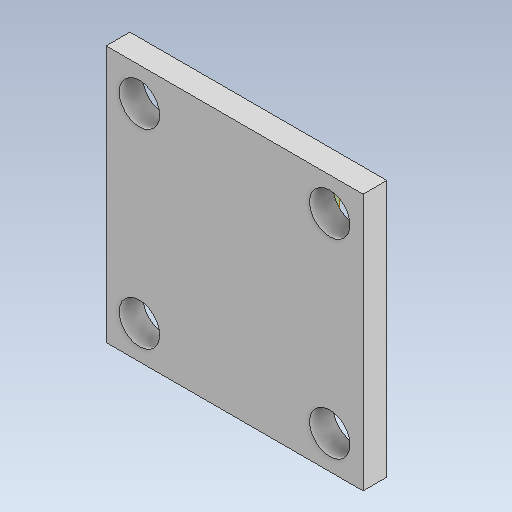
# Autodesk Inventor part: Magazin_1_trichter
Saved by Autodesk Inventor 2025.2 (Build 292293000, 293)
## iProperties
Created: 2025-06-10
Part Number: Magazin_1_trichter
Material: Generisch
Document SubType Name: Modeling
Designer: maria
Density: 1 g/cm^3
Appearance: Vorgabe
Author: maria
## iProperties of the stored document Magazin_1_3D-Druck.ipt
Created: 2025-06-10
Part Number: Magazin_1_3D-Druck
Material: Generisch
Document SubType Name: Modeling
Designer: maria
Density: 1 g/cm^3
Appearance: Vorgabe
Author: maria
Autodesk Inventor part; units mm, degrees
ref_plane "YZ Plane" through (0, 0, 0) normal (1, 0, 0) x (0, 1, 0)
ref_plane "XZ Plane" through (0, 0, 0) normal (0, 1, 0) x (-1, 0, 0)
ref_plane "XY Plane" through (0, 0, 0) normal (0, 0, 1) x (1, 0, 0)
sketch "Skizze1" plane through (0, 0, 0) normal (0, 1, 0) x (-1, 0, 0)
  line L0 (0, 0) -> (12, 0)
  line L1 (12, 0) -> (12, -16)
  line L2 (12, -16) -> (0, -16)
  line L3 (0, -16) -> (0, 0)
  line L4 (17, 5) -> (17, -21)
  line L5 (-5, -21) -> (-5, 5)
  line L6 (-1, 1) -> (13, 1)
  line L7 (13, 1) -> (13, -17)
  line L8 (13, -17) -> (-1, -17)
  line L9 (-1, -17) -> (-1, 1)
  line L10 (1.75, -1.75) -> (10.25, -1.75)
  line L11 (10.25, -1.75) -> (10.25, -14.25)
  line L12 (10.25, -14.25) -> (1.75, -14.25)
  line L13 (1.75, -14.25) -> (1.75, -1.75)
  line L14 (0.75, -0.75) -> (11.25, -0.75)
  line L15 (11.25, -0.75) -> (11.25, -15.25)
  line L16 (11.25, -15.25) -> (0.75, -15.25)
  line L17 (0.75, -15.25) -> (0.75, -0.75)
  line L18 (15.25, 5.25) -> (-3.25, 5.25)
  line L19 (-3.25, 5.25) -> (-3.25, -21.25)
  line L20 (-3.25, -21.25) -> (15.25, -21.25)
  line L21 (15.25, -21.25) -> (15.25, 5.25)
  line L22 (16.25, 6.25) -> (-4.25, 6.25)
  line L23 (-4.25, 6.25) -> (-4.25, -22.25)
  line L24 (-4.25, -22.25) -> (16.25, -22.25)
  line L25 (16.25, -22.25) -> (16.25, 6.25)
  point P0 (6, 0)
  point P1 (6, 5)
  point P2 (6, -16)
  point P3 (12, -8)
  point P4 (6, -1.75)
  point P5 (6, -14.25)
  point P6 (10.25, -8)
  point P7 (1.75, -8)
  point P8 (6, -21.25)
  dimension "d0" = 16
  dimension "d1" = 12
  dimension "d2" = 5
  dimension "d3" = 5
  dimension "d56" = 1
  dimension "d57" = 1
  dimension "d58" = 1
  dimension "d60" = 1.75
  dimension "d61" = 1.75
  dimension "d63" = 8.5
  dimension "d64" = 1
  dimension "d65" = 1
  dimension "d67" = 1
  dimension "d69" = 12.5
  dimension "d70" = 1
  dimension "d71" = 1.75
  dimension "d72" = 1.75
  dimension "d74" = 7
  dimension "d76" = 7
  dimension "d77" = 5
  dimension "d78" = 5
  dimension "d80" = 1
  dimension "d81" = 1
  dimension "d82" = 1
  dimension "d83" = 1
  constraints: 52 end point, 13 parallel, 8 midpoint, 6 horizontal, 6 perpendicular
  measures "d0" distance of L0.end L1.end
  measures "d1" distance of L1.end L2.end
  measures "d2" distance between parallel lines of L4 L1
  measures "d3" distance between parallel lines of L5 L3
  measures "d56" distance between parallel lines of L0 L6
  measures "d57" distance from line of L7 point (12, -8)
  measures "d58" distance between parallel lines of L8 L2
  measures "d60" distance of point (6, 0) point (6, -1.75)
  measures "d61" distance from line of L2 point (6, -14.25)
  measures "d63" distance of point (10.25, -8) point (1.75, -8)
  measures "d64" distance between parallel lines of L10 L14
  measures "d65" distance between parallel lines of L15 L11
  measures "d67" distance between parallel lines of L13 L17
  measures "d69" distance between parallel lines of L10 L12
  measures "d70" distance between parallel lines of L16 L12
  measures "d71" distance between parallel lines of L1 L11
  measures "d72" distance between parallel lines of L3 L13
  measures "d74" distance from line of point (6, -21.25) L12
  measures "d76" distance between parallel lines of L18 L10
  measures "d77" distance between parallel lines of L19 L13
  measures "d78" distance between parallel lines of L21 L11
  measures "d80" distance between parallel lines of L22 L18
  measures "d81" distance between parallel lines of L24 L20
  measures "d82" distance between parallel lines of L19 L23
  measures "d83" distance between parallel lines of L25 L21
ref_plane "Arbeitsebene1" through (0, 0, 0) normal (0, -1, 0) x (1, 0, 0)
sketch "Skizze2" plane through (0, 0, 0) normal (0, -1, 0) x (1, 0, 0)
  line L0 (21, 19) -> (-33, 19)
  line L1 (-33, 19) -> (-33, -35)
  line L2 (-33, -35) -> (21, -35)
  line L3 (21, -35) -> (21, 19)
  line L4 (-17, -21) -> (-17, 5) projected
  line L5 (5, -21) -> (-17, -21) projected
  line L6 (5, 5) -> (5, -21) projected
  line L7 (-17, 5) -> (5, 5) projected
  point P0 (0, 0)
  dimension "d11" = 16
  dimension "d12" = 14
  dimension "d13" = 16
  dimension "d14" = 14
  dimension "d35" = 54
  dimension "d36" = 54
  constraints: 8 end point, 2 parallel, 1 horizontal, 1 perpendicular
  measures "d11" distance between parallel lines of L4 L1
  measures "d12" distance between parallel lines of L2 L5
  measures "d13" distance between parallel lines of L3 L6
  measures "d14" distance between parallel lines of L0 L7
  measures "d35" distance of L0.end L1.end
  measures "d36" distance of L0.start L0.end
extrude "Extrusion2" add sketch "Skizze2" along normal blind 5 contours L3 L2 L1 L0 | L4 L7 L6 L5
ref_plane "Arbeitsebene2" through (0, 0, 0) normal (0, 1, 0) x (1, 0, 0)
sketch "Skizze4" plane through (0, 0, 0) normal (0, 1, 0) x (1, 0, 0)
  line L0 (21, 35) -> (21, -19) projected
  line L1 (-33, 35) -> (21, 35) projected
  line L2 (21, -19) -> (-33, -19) projected
  line L3 (-33, -19) -> (-33, 35) projected
  point P0 (0, 0)
  point P1 (14, 28)
  point P2 (14, -12)
  point P3 (-26, -12)
  point P4 (-26, 28)
  dimension "d44" = 7
  dimension "d45" = 7
  dimension "d46" = 7
  dimension "d47" = 7
  dimension "d48" = 7
  dimension "d49" = 7
  dimension "d50" = 7
  dimension "d51" = 7
  dimension "d52" = 40
  dimension "d53" = 40
  dimension "d54" = 40
  dimension "d55" = 40
  measures "d44" distance from line of L0 point (14, 28)
  measures "d45" distance from line of L1 point (14, 28)
  measures "d46" distance from line of L0 point (14, -12)
  measures "d47" distance from line of L2 point (14, -12)
  measures "d48" distance from line of L3 point (-26, -12)
  measures "d49" distance from line of L2 point (-26, -12)
  measures "d50" distance from line of L1 point (-26, 28)
  measures "d51" distance from line of L3 point (-26, 28)
  measures "d52" distance of point (14, -12) point (14, 28)
  measures "d53" distance of point (-26, 28) point (14, 28)
  measures "d54" distance of point (-26, -12) point (-26, 28)
  measures "d55" distance of point (14, -12) point (-26, -12)
hole "Bohrung1" at (14, 0, -28) at (14, 0, 12) at (-26, 0, 12) at (-26, 0, -28) direction (0, -1, 0) diameter 8.5 depth 5
extrude "Extrusion4" add sketch "Skizze1" along normal blind 4 contours L25 L24 L23 L22
